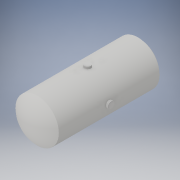
# Autodesk Inventor part: air canister
Saved by Autodesk Inventor 2018 (Build 220112000, 112)
## iProperties
Created: 2017-05-02
Part Number: air canister
Material: Generic
Document SubType Name: Modeling
Designer: gsegs
Density: 1 g/cm^3
Appearance: Default
Author: gsegs
Autodesk Inventor part; units mm, degrees
ref_plane "XZ Plane" through (0, 0, 0) normal (0, 1, 0) x (-1, 0, 0)
ref_plane "XY Plane" through (0, 0, 0) normal (0, 0, 1) x (1, 0, 0)
sketch "Sketch1" plane through (0, 0, 0) normal (0, 0, 1) x (1, 0, 0)
  circle A0 centre (0, 0) radius 84.1375
  dimension "d0" = 168.275
  constraints: 1 centre point, 1 coincident
  measures "d0" diameter of A0
extrude "Extrusion1" add sketch "Sketch1" along normal blind 457.2
sketch "Sketch2" plane through (0, 0, 0) normal (1, 0, 0) x (0, 1, 0)
  arc A0 (0, 0) -> (84.1375, 33.3375) centre (0, 122.8423) ccw
  line L0 (0, -110.2072) -> (0, 551.7679) projected
  line L1 (84.1375, 0) -> (84.1375, 457.2) projected
  line L2 (84.1375, 457.2) -> (-84.1375, 457.2) projected
  arc A1 (84.1375, 423.8625) -> (0, 457.2) centre (0, 334.3577) ccw
  line L3 (-84.1375, 0) -> (84.1375, 0) projected
  dimension "d3" = 390.525
  dimension "d4" = 33.3375
  dimension "d5" = 33.3375
  constraints: 4 point on circle, 2 centre point, 2 line through centre, 2 point on line, 1 midpoint
  measures "d3" distance of A0.end A1.start
  measures "d4" distance from line of L2 A1.start
  measures "d5" distance from line of L3 A0.end
revolve "Revolution1" cut sketch "Sketch2" angle 360 about axis through (0, 0, -10) along (0, 0, 1) contours A0 L1 L3 | L2 L1 A1
sketch "Sketch3" plane through (0, 0, 0) normal (0, 0, 1) x (1, 0, 0)
  circle A0 centre (0, 0) radius 16.0528
  dimension "d7" = 32.1056
  constraints: 1 centre point, 1 coincident
  measures "d7" diameter of A0
extrude "Extrusion2" add sketch "Sketch3" along normal blind 32.1056 and the other way blind 11.684
ref_plane "Work Plane1" through (84.1375, 0, 0) normal (1, 0, 0) x (0, 1, 0)
sketch "Sketch4" plane through (84.1375, 0, 0) normal (1, 0, 0) x (0, 1, 0)
  line L0 (84.1375, 33.3375) -> (-84.1375, 33.3375) construction
  line L1 (-84.1375, 423.8625) -> (84.1375, 423.8625) construction
  line L2 (0, 423.8625) -> (0, 33.3375) construction
  circle A0 centre (0, 228.6) radius 12.7
  point P0 (0, 0)
  dimension "d12" = 25.4
  constraints: 3 midpoint, 2 end point, 1 centre point
  measures "d12" diameter of A0
extrude "Extrusion3" add sketch "Sketch4" along normal blind 7.62 and the other way blind 7.62
pattern_circular "Circular Pattern1" count 2 over 90 about axis through (0, 0, -10) along (0, 0, 1) of "Extrusion3"
equation "\"d8\" = d7"
body "Solid1"
